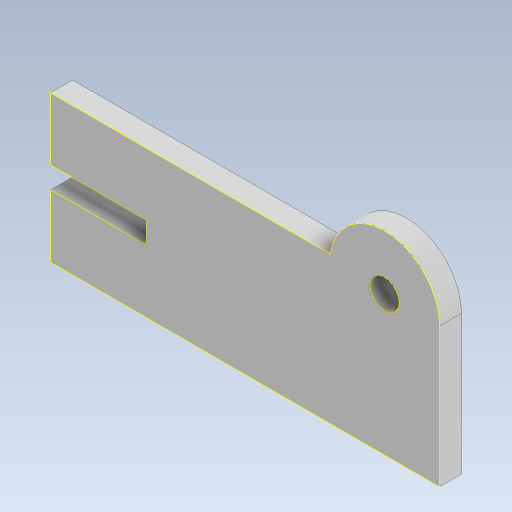
# Autodesk Inventor part: 零件7
Saved by Autodesk Inventor 2023 (Build 270158000, 158)
## iProperties
Created: 2023-05-12
Part Number: 零件7
Material: 一般
Document SubType Name: Modeling
Designer: Johnny Jou
Density: 1 g/cm^3
Appearance: 預設
Author: Johnny Jou
Autodesk Inventor part; units mm, degrees
ref_plane "YZ Plane" through (0, 0, 0) normal (1, 0, 0) x (0, 1, 0)
ref_plane "XZ Plane" through (0, 0, 0) normal (0, 1, 0) x (-1, 0, 0)
ref_plane "XY Plane" through (0, 0, 0) normal (0, 0, 1) x (1, 0, 0)
sketch "草圖1" plane through (0, 0, 0) normal (0, 0, 1) x (1, 0, 0)
  line L0 (0, 0) -> (38, 0)
  line L1 (38, -20) -> (0, -20)
  line L2 (0, -20) -> (0, 0)
  line L3 (0, -8.525) -> (13, -8.525)
  line L4 (13, -8.525) -> (13, -11.475)
  line L5 (13, -11.475) -> (0, -11.475)
  line L6 (0, -11.475) -> (0, -8.525)
  line L7 (38, 0) -> (60, 0)
  line L8 (38, 0) -> (38, -20)
  line L9 (38, -20) -> (53, -20)
  line L10 (53, -20) -> (53, 6.475)
  line L11 (53, 6.475) -> (38, 6.475)
  line L12 (38, 6.475) -> (38, -20)
  circle A0 centre (45.5, -1.025) radius 1.975
  circle A1 centre (45.5, -1.025) radius 7.5
  point P0 (13, -10)
  point P1 (0, -10)
  point P2 (38, 0)
  point P3 (38.0704, 0)
  point P4 (53, -1.025)
  dimension "d0" = 20
  dimension "d2" = 13
  dimension "d3" = 2.95
  dimension "d4" = 0
  dimension "d7" = 38
  dimension "d9" = 3.95
  dimension "d12" = 15
  constraints: 26 end point, 5 parallel, 4 horizontal, 4 tangent, 3 perpendicular, 2 centre point, 2 midpoint, 1 coincident, 1 point on line
  measures "d0" distance between parallel lines of L1 L0
  measures "d2" distance of L3.start L3.end
  measures "d3" distance of L3.end L4.end
  measures "d4" vertical distance of point (13, -10) point (0, -10)
  measures "d7" distance between parallel lines of L2 L8
  measures "d9" diameter of A0
  measures "d12" distance between parallel lines of L10 L12
extrude "擠出1" add sketch "草圖1" along normal blind 3 contours L0 L8 L1 L2 L5 L4 L3 | L7 A1 L8 | A1 L7 A0 | L7 A0 A1 | A1 L10 L9 L8
sketch "草圖2" plane through (0, 0, 3) normal (0, 0, 1) x (1, 0, 0)
  line L0 (0, -20) -> (53, -20) projected
  line L1 (53, -20) -> (53, -1.025) projected
  line L2 (38.0704, 0) -> (0, 0) projected
  line L3 (0, 0) -> (0, -8.525) projected
  circle A0 centre (45.5, -1.025) radius 1.975 projected
  line L4 (0, -8.525) -> (13, -8.525) projected
  line L5 (13, -8.525) -> (13, -11.475) projected
  line L6 (13, -11.475) -> (0, -11.475) projected
  line L7 (0, -11.475) -> (0, -20) projected
  arc A1 (53, -1.025) -> (38.0704, 0) centre (45.5, -1.025) ccw projected
